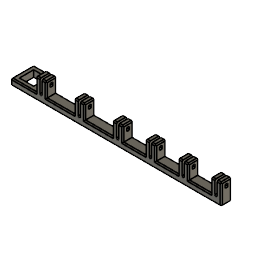
Idler Pulley Tool Holder (Autodesk Fusion 360 design; units mm, degrees)
Autodesk Fusion 360 part; units mm, degrees
box "BoxPrimitive1" add length 9.525 width 19.05 height 9.525 placed x (0, -1, 0) y (1, 0, 0) z (0, 0, 1) at (-19.05, 12.3721, 0) makes body 1
sketch "Sketch2" plane through (0, 0, 9.525) normal (0, 0, 1) x (-1, 0, 0)
  line L0 (19.05, -2.8471) -> (0, -2.8471)
  line L1 (0, -2.8471) -> (0, -12.3721)
  line L2 (0, -12.3721) -> (19.05, -12.3721)
  line L3 (19.05, -12.3721) -> (19.05, -2.8471)
  line L4 (19.05, -12.3721) -> (19.05, -2.8471)
  line L5 (19.05, -7.6096) -> (8.1976, -7.6096) construction
  line L6 (7, -8.6096) -> (19.05, -8.6096)
  line L7 (7, -6.6096) -> (19.05, -6.6096)
  arc A0 (7, -6.6096) -> (7, -8.6096) centre (7, -7.6096) ccw
  dimension "d12" = 6
  dimension "d13" = 2
  constraint midpoint L4 L5.start
  constraint perpendicular L3 L5
  constraint coincident L4 L6.end
  constraint perpendicular L4 L6
  constraint symmetric L5 L6.start L7.start
  constraint symmetric L5 L6.end L7.end
  constraint tangent L7 A0
  measures "d12" distance of L1 A0
  measures "d13" distance of L6 L7
extrude "Extrude1" cut sketch "Sketch2" against normal blind 9.525 contours L3 L4 L6 L7 A0 bodies 1
chamfer "Chamfer1" distance 1 angle 45 4 edges at (-9.525, 12.3721, 9.525) (-9.525, 12.3721, 0) (-9.525, 2.8471, 0) (-9.525, 2.8471, 9.525) on bodies 1
sketch "Sketch3" plane through (-19.05, 0, 0) normal (-1, 0, 0) x (0, -1, 0)
  line L0 (-12.3721, 1) -> (-11.3721, 0)
  line L1 (-11.3721, 0) -> (-8.6096, 0)
  line L2 (-8.6096, 0) -> (-8.6096, 9.525)
  line L3 (-8.6096, 9.525) -> (-11.3721, 9.525)
  line L4 (-11.3721, 9.525) -> (-12.3721, 8.525)
  line L5 (-12.3721, 8.525) -> (-12.3721, 1)
  line L6 (-12.3721, 8.525) -> (-12.3721, 1)
  line L7 (-12.3721, 4.7625) -> (-13.3721, 4.7625) construction
  line L8 (-13.3721, 4.9625) -> (-12.3721, 5.9625)
  line L9 (-13.3721, 4.5625) -> (-12.3721, 3.5625)
  line L10 (-13.3721, 4.9625) -> (-13.3721, 4.5625)
  dimension "d9" = 45
  dimension "d10" = 1
  dimension "d11" = 0.4
  constraint midpoint L5 L7.start
  constraint perpendicular L5 L7
  constraint coincident L5 L8.end
  constraint symmetric L7 L8.end L9.end
  constraint perpendicular L7 L10
  constraint coincident L10 L7.end
  constraint symmetric L7 L8 L9
  measures "d9" angle of L6 L9
  measures "d10" distance of L7.start L7.end
  measures "d11" distance of L8.start L9.start
extrude "Extrude2" add sketch "Sketch3" against normal blind 3 from surface at -3 contours L5 L6 L8 L9 L10 bodies 1
chamfer "Chamfer2" distance 1 angle 45 2 edges at (-16.05, 13.3721, 4.7625) (-13.05, 13.3721, 4.7625) on bodies 1
chamfer "Chamfer3" distance 1 angle 45 10 edges at (-19.05, 12.3721, 4.7625) (-19.05, 9.9909, 9.525) (-19.05, 5.2284, 9.525) (-19.05, 2.8471, 4.7625) (-19.05, 5.2284, 0) (-19.05, 9.9909, 0) (0, 7.6096, 9.525) (0, 2.8471, 4.7625) (0, 7.6096, 0) (0, 12.3721, 4.7625) on bodies 1
sketch "Sketch1" plane through (0, 0, 0) normal (0, 0, 1) x (1, 0, 0) in component "Base"
  line L0 (0, 0) -> (200.85, 0)
  line L1 (200.85, 0) -> (200.85, 25.4)
  line L2 (200.85, 25.4) -> (0, 25.4)
  line L3 (0, 25.4) -> (0, 0)
  line L4 (0, 12.7) -> (10.35, 12.7) construction
  line L5 (4, 19.05) -> (16.7, 19.05)
  line L6 (16.7, 19.05) -> (16.7, 6.35)
  line L7 (16.7, 6.35) -> (4, 6.35)
  line L8 (4, 6.35) -> (4, 19.05)
  line L9 (4, 19.05) -> (16.7, 6.35) construction
  line L10 (16.7, 19.05) -> (4, 6.35) construction
  point P0 (10.35, 12.7)
  dimension "d19" = 12.7
  dimension "d20" = 12.7
  dimension "d21" = 4
  dimension "d22" = 25.4
  dimension "d23" = 184.15
  constraint horizontal L0
  constraint vertical L1
  constraint horizontal L2
  constraint vertical L3
  constraint coincident L0.start L3.end
  constraint midpoint L3 L4.start
  constraint perpendicular L3 L4
  constraint horizontal L5
  constraint perpendicular L5 L6
  constraint parallel L5 L7
  constraint parallel L6 L8
  constraint coincident L9 P0
  constraint coincident L10 P0
  constraint coincident P0 L4.end
  measures "d19" distance of L5.end L6.end
  measures "d20" distance of L5.start L5.end
  measures "d21" distance of L3 L8
  measures "d22" distance of L0 L2
  measures "d23" distance of L1 L6
extrude "Extrude1'" add sketch "Sketch1" along normal blind 8 separate body makes body 2 in component "Base"
fillet "Fillet1" radius 2 4 edges at (0, 0, 4) (0, 25.4, 4) (200.85, 0, 4) (200.85, 25.4, 4) on bodies 2 in component "Base"
copy_body "CopyPasteBodies1" bodies 1 makes body 3 in component "Idler Pulley Tool Holder"
move_body "Move1" bodies 3 to x (0, 0, -1) y (0, 1, 0) z (1, 0, 0) at (-19.05, 0, -19.05) in component "Idler Pulley Tool Holder"
move_body "Move2" bodies 3 to x (0, -1, 0) y (1, 0, 0) z (0, 0, 1) at (-21.8971, -6.6779, 0) in component "Idler Pulley Tool Holder"
pattern_linear "R-Pattern1" count 1 spacing 35 along (0, -1, 0) count 3 spacing 35 along (1, 0, 0) of bodies 3 makes body 4 at (15.95, 6.3555, -12.3667) makes body 5 at (50.95, 6.3555, -12.3667) in component "Idler Pulley Tool Holder"
pattern_linear "R-Pattern2" count 4 spacing 30 along (1, 0, 0) of bodies 5 makes body 6 at (80.95, 6.3555, -12.3667) makes body 7 at (110.95, 8.8638, -12.3667) makes body 8 at (140.95, 6.3555, -12.3667) in component "Idler Pulley Tool Holder"
sketch "Sketch2 (2)" plane through (0, 0, -19.05) normal (0, 0, -1) x (1, 0, 0) in component "Idler Pulley Tool Holder"
  line L0 (164.475, -11.3721) -> (164.475, -3.8471)
  line L1 (164.475, -3.8471) -> (156.95, -3.8471)
  line L2 (156.95, -3.8471) -> (156.95, -11.3721)
  line L3 (156.95, -11.3721) -> (164.475, -11.3721)
  line L4 (-19.05, -3.8471) -> (-19.05, -11.3721) construction
  line L5 (-42.05, -2.8471) -> (149.475, -2.8471)
  line L6 (149.475, -12.3721) -> (-21.05, -12.3721)
  line L7 (-21.05, -12.3721) -> (-21.05, -23.8471)
  line L8 (-21.05, -23.8471) -> (-42.05, -23.8471)
  line L9 (-42.05, -23.8471) -> (-42.05, -2.8471)
  line L10 (-38.05, -6.8471) -> (-25.05, -6.8471)
  line L11 (-25.05, -6.8471) -> (-25.05, -19.8471)
  line L12 (-25.05, -19.8471) -> (-38.05, -19.8471)
  line L13 (-38.05, -19.8471) -> (-38.05, -6.8471)
  line L14 (149.475, -12.3721) -> (150.475, -11.3721)
  line L15 (150.475, -11.3721) -> (150.475, -3.8471)
  line L16 (150.475, -3.8471) -> (149.475, -2.8471)
  line L17 (59.475, -11.3721) -> (59.475, -3.8471)
  line L18 (59.475, -3.8471) -> (51.95, -3.8471)
  line L19 (51.95, -3.8471) -> (51.95, -11.3721)
  line L20 (51.95, -11.3721) -> (59.475, -11.3721)
  point P0 (-18.05, -2.8471)
  point P1 (-18.05, -12.3721)
  point P2 (150.475, -3.8471)
  point P3 (150.475, -11.3721)
  dimension "d39" = 13
  dimension "d40" = 6
  dimension "d41" = 4
  dimension "d42" = 4
  dimension "d44" = 4
  dimension "d45" = 4
  dimension "d46" = 13
  constraint perpendicular L6 L7
  constraint perpendicular L7 L8
  constraint perpendicular L5 L9
  constraint coincident L5.start L9.end
  constraint horizontal L10
  constraint vertical L11
  constraint horizontal L12
  constraint vertical L13
  constraint coincident P0 L5
  constraint coincident L6.start L14.start
  constraint coincident P3 L14.end
  constraint coincident P2 L15.end
  constraint coincident L5.end L16.end
  measures "d39" distance of L11.end L12.end
  measures "d40" distance of L4 L11
  measures "d41" distance of L9 L13
  measures "d42" distance of L5 L10
  measures "d44" distance of L7 L11
  measures "d45" distance of L8 L12
  measures "d46" distance of L10.start L12.end
extrude "Extrude1''" add sketch "Sketch2 (2)" against normal blind 6 contours L5 L6 L7 L8 L9 L14 L15 L16 | L17 L18 L19 L20 bodies 3 4 5 6 7 8 in component "Idler Pulley Tool Holder"
chamfer "Chamfer2'" distance 3 angle 45 1 edges at (-21.05, 12.3721, -16.05) on bodies 3 in component "Idler Pulley Tool Holder"
chamfer "Chamfer1'" distance 1 angle 45 27 edges at (53.7125, 2.8471, -19.05) (65.7125, 12.3721, -19.05) (150.475, 7.6096, -19.05) (149.975, 11.8721, -19.05) (149.975, 3.3471, -19.05) (-42.05, 13.3471, -19.05) (-31.55, 23.8471, -19.05) (-21.05, 19.6096, -19.05) (-42.05, 2.8471, -16.05) (-42.05, 23.8471, -16.05) (-21.05, 23.8471, -16.05) (-19.55, 13.8721, -19.05) (-19.55, 13.8721, -13.05) (-21.05, 19.6096, -13.05) (-31.55, 23.8471, -13.05) (-30.05, 2.8471, -13.05) (-42.05, 13.3471, -13.05) (38.2125, 12.3721, -13.05) (38.2125, 2.8471, -13.05) (3.2125, 2.8471, -13.05) (3.2125, 12.3721, -13.05) (130.7125, 2.8471, -13.05) (130.7125, 12.3721, -13.05) (100.7125, 12.3721, -13.05) (100.7125, 2.8471, -13.05) (70.7125, 12.3721, -13.05) (70.7125, 2.8471, -13.05) on bodies 3 in component "Idler Pulley Tool Holder"
component "Base" placed x (1, 0, 0) y (0, 1, 0) z (0, 0, 1) at (0, 0, 0)
component "Idler Pulley Tool Holder" placed x (1, 0, 0) y (0, 1, 0) z (0, 0, 1) at (0, 0, 0)
equation "d1 = ( 3 / 8 ) * 1 in"
equation "d2 = ( 3 / 8 ) * 2 in"
equation "d3 = ( 3 / 8 ) * 1 in"
equation "d19 = 0.5 * 1 in"
equation "d20 = d19"
equation "d23 = 7.25 * 1 in"
equation "d41 = d42"
equation "d44 = d42"
equation "d45 = d42"
equation "d46 = d39"
named bodies: "Primitive socket holder", "BaseV2", "Idler Pulley Tool Holder"
